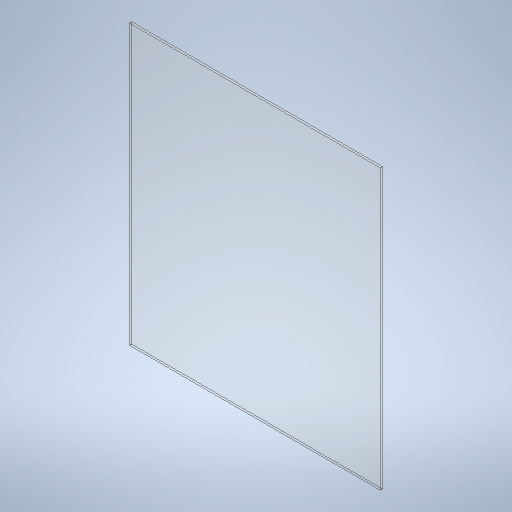
# Autodesk Inventor part: workbench door
Saved by Autodesk Inventor 2025 (Build 290162010, 162A)
## iProperties
Created: 2024-06-17
Part Number: workbench door
Material: Polycarbonate, Clear
Document SubType Name: Modeling
Designer: Alan Thomas
Mass: 9109.9 g
Surface Area: 19291.1 cm^2
Volume: 7591.58 cm^3
Density: 1.2 g/cm^3
Appearance: Polycarbonate - Clear
Author: Alan Thomas
Autodesk Inventor part; units mm, degrees
ref_plane "YZ Plane" through (0, 0, 0) normal (1, 0, 0) x (0, 1, 0)
ref_plane "XZ Plane" through (0, 0, 0) normal (0, 1, 0) x (-1, 0, 0)
ref_plane "XY Plane" through (0, 0, 0) normal (0, 0, 1) x (1, 0, 0)
sketch "Sketch1" plane through (0, 0, 0) normal (0, 0, 1) x (1, 0, 0)
  line L0 (0, 0) -> (924, 0)
  line L1 (924, 0) -> (924, 1027)
  line L2 (924, 1027) -> (0, 1027)
  line L3 (0, 1027) -> (0, 0)
  dimension "d0" = 924
  dimension "d1" = 1027
  constraints: 8 end point, 2 parallel, 1 horizontal, 1 perpendicular
  measures "d0" distance of L2.end L1.end
  measures "d1" distance of L1.end L0.end
extrude "Extrusion1" add sketch "Sketch1" along normal blind 8
body "Solid1"
